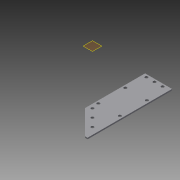
# Autodesk Inventor part: Extender Mounting Plate
Saved by Autodesk Inventor 2013 (Build 170138000, 138)
## iProperties
Created: 2013-01-19
Part Number: Extender Mounting Plate
Material: Generic
Document SubType Name: Modeling
Designer: actoennies
Density: 1 g/cm^3
Author: actoennies
Autodesk Inventor part; units mm, degrees
ref_plane "YZ Plane" through (0, 0, 0) normal (1, 0, 0) x (0, 1, 0)
ref_plane "XZ Plane" through (0, 0, 0) normal (0, 1, 0) x (-1, 0, 0)
ref_plane "XY Plane" through (0, 0, 0) normal (0, 0, 1) x (1, 0, 0)
sketch "Sketch1" plane through (0, 0, 0) normal (0, 1, 0) x (-1, 0, 0)
  circle A0 centre (0, 0) radius 152.4 construction
  circle A1 centre (0, 0) radius 203.2 construction
  line L0 (0, 0) -> (0, -94.5056)
  line L1 (0, 0) -> (255.4804, -255.4804) construction
  circle A2 centre (152.4, 0) radius 3.3782
  circle A3 centre (203.2, 0) radius 3.3782
  circle A4 centre (107.7631, -107.7631) radius 3.3782
  circle A5 centre (143.6841, -143.6841) radius 3.3782
  line L2 (250.9903, -259.9706) -> (8.0112, -16.9915)
  line L3 (143.6841, -152.6644) -> (152.6644, -143.6841)
  line L4 (98.7828, -107.7631) -> (107.7631, -98.7828)
  line L5 (146.05, 6.35) -> (209.55, 6.35)
  line L6 (209.55, 6.35) -> (209.55, -6.35)
  line L7 (146.05, -6.35) -> (146.05, 6.35)
  line L8 (152.6644, -143.6841) -> (209.55, -6.35)
  line L9 (146.05, -6.35) -> (107.7631, -98.7828)
  circle A6 centre (175.8001, -60.9582) radius 3.3782
  circle A7 centre (157.3663, -122.0546) radius 3.3782
  circle A8 centre (140.6003, -46.378) radius 3.3782
  circle A9 centre (116.2999, -105.0443) radius 3.3782
  dimension "d34" = 304.8
  dimension "d36" = 406.4
  dimension "d38" = 45
  dimension "d40" = 6.7564
  dimension "d41" = 6.7564
  dimension "d42" = 6.7564
  dimension "d43" = 6.7564
  dimension "d44" = 6.35
  dimension "d45" = 6.35
  dimension "d46" = 6.35
  dimension "d48" = 6.35
  dimension "d49" = 6.35
  dimension "d51" = 6.35
  dimension "d52" = 6.35
  dimension "d53" = 157.5
  dimension "d58" = 6.7564
  dimension "d59" = 6.7564
  dimension "d64" = 6.7564
  dimension "d70" = 6.7564
  dimension "d72" = 63.5
  constraints: 20 end point, 10 centre point, 4 point on circle, 4 point on line, 3 parallel, 3 perpendicular, 2 coincident, 1 vertical
  measures "d34" diameter of A0
  measures "d36" diameter of A1
  measures "d38" angle of L1 L0
  measures "d40" diameter of A2
  measures "d41" diameter of A3
  measures "d42" diameter of A4
  measures "d43" diameter of A5
  measures "d44" distance between parallel lines of L1 L2
  measures "d45" distance from line of A5.centre L3
  measures "d46" distance from line of L4 A4.centre
  measures "d48" distance from line of L5 A2.centre
  measures "d49" distance from line of L6 A3.centre
  measures "d51" distance from line of L5 A3.centre
  measures "d52" distance from line of A2.centre L7
  measures "d53" angle of L7 L9
  measures "d58" diameter of A6
  measures "d59" diameter of A7
  measures "d64" diameter of A8
  measures "d70" diameter of A9
  measures "d72" distance of A8.centre A9.centre
ref_plane "Work Plane1" through (0, 3.175, 0) normal (0, 1, 0) x (1, 0, 0)
extrude "Extrusion5" add sketch "Sketch1" along normal blind 3.175
body "Solid1"
